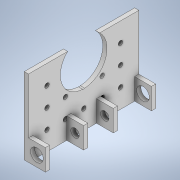
# Autodesk Inventor part: plateForAzimuthKnobs
Saved by Autodesk Inventor 2022.2 (Build 262287010, 287A)
## iProperties
Created: 2022-09-17
Part Number: plateForAzimuthKnobs
Material: Generic
Document SubType Name: Modeling
Designer: robst
Density: 1 g/cm^3
Appearance: Default
Author: robst
Autodesk Inventor part; units mm, degrees
ref_plane "YZ Plane" through (0, 0, 0) normal (1, 0, 0) x (0, 1, 0)
ref_plane "XZ Plane" through (0, 0, 0) normal (0, 1, 0) x (-1, 0, 0)
ref_plane "XY Plane" through (0, 0, 0) normal (0, 0, 1) x (1, 0, 0)
sketch "Sketch1" plane through (0, 0, 0) normal (1, 0, 0) x (0, 1, 0)
  line L0 (-57.2668, 82.55) -> (-57.2668, -82.55)
  line L1 (-57.2668, -82.55) -> (57.2668, -82.55)
  line L2 (57.2668, -82.55) -> (57.2668, 82.55)
  line L3 (57.2668, 82.55) -> (-57.2668, 82.55)
  line L4 (-57.2668, 82.55) -> (57.2668, -82.55) construction
  line L5 (-57.2668, -82.55) -> (57.2668, 82.55) construction
  line L6 (57.2668, 0) -> (-57.2668, 0) construction
  circle A0 centre (31.8668, 0) radius 34.925
  line L7 (-31.8668, 82.55) -> (-31.8668, -82.55) construction
  point P0 (0, 0)
  point P1 (57.2668, -23.9707)
  point P2 (57.2668, 23.9707)
  dimension "d0" = 165.1
  dimension "d1" = 25.4
  dimension "d2" = 69.85
  dimension "d3" = 63.7337
  dimension "d4" = 25.4
  constraints: 16 end point, 4 midpoint, 3 point on line, 2 parallel, 2 perpendicular, 1 centre point, 1 vertical
  measures "d0" distance of L1.end L2.end
  measures "d1" distance from line of A0.centre L2
  measures "d2" diameter of A0
  measures "d3" distance from line of L7 A0.centre
  measures "d4" distance between parallel lines of L7 L0
extrude "Extrusion1" add sketch "Sketch1" against normal blind 6.35 contours L3 L2 A0 L1 L0
sketch "Sketch2" plane through (0, 0, 0) normal (1, 0, 0) x (0, 0, -1)
  line L0 (82.55, -57.2668) -> (-82.55, -57.2668) projected
  line L1 (-82.55, -57.2668) -> (-76.2, -57.2668)
  line L2 (-76.2, -57.2668) -> (-76.2, -25.5168)
  line L3 (-76.2, -25.5168) -> (-82.55, -25.5168)
  line L4 (-82.55, -25.5168) -> (-82.55, -57.2668)
  line L5 (82.55, -57.2668) -> (76.2, -57.2668)
  line L6 (76.2, -57.2668) -> (76.2, -25.5168)
  line L7 (76.2, -25.5168) -> (82.55, -25.5168)
  line L8 (82.55, -25.5168) -> (82.55, -57.2668)
  point P0 (0, 0)
  point P1 (76.2, -57.2668)
  dimension "d7" = 6.35
  dimension "d8" = 6.35
  dimension "d15" = 31.75
  constraints: 16 end point, 4 parallel, 2 horizontal, 2 perpendicular, 1 collinear
  measures "d7" distance between parallel lines of L2 L4
  measures "d8" distance between parallel lines of L6 L8
  measures "d15" distance of L3.end L0.end
extrude "Extrusion2" add sketch "Sketch2" along normal blind 25.2001
sketch "Sketch4" plane through (-6.35, 57.2668, 82.55) normal (0, 0, 1) x (1, 0, 0)
  line L0 (31.5501, -82.7837) -> (31.5501, -114.5337) construction
  line L1 (31.5501, -98.6587) -> (0, -98.6587) construction
  line L2 (0, 0) -> (0, -114.5337) construction
  circle A0 centre (18.8501, -98.6587) radius 9.525
  point P0 (6.35, -57.2668)
  dimension "d11" = 18.8501
  dimension "d12" = 19.05
  constraints: 2 end point, 2 point on line, 1 centre point, 1 horizontal, 1 midpoint
  measures "d11" distance from line of A0.centre L2
  measures "d12" diameter of A0
extrude "Extrusion3" cut sketch "Sketch4" against normal up to surface (6.35 mm away)
sketch "Sketch5" plane through (-6.35, 0, 0) normal (-1, 0, 0) x (0, 0, 1)
  line L0 (-82.55, 57.2668) -> (-82.55, -57.2668) projected
  line L1 (-82.55, -57.2668) -> (82.55, -57.2668) projected
  point P0 (0, 0)
  point P1 (-55.0333, -28.6334)
  dimension "d23" = 27.5167
  dimension "d24" = 28.6334
  measures "d23" distance from line of point (-55.033, -28.633) L0
  measures "d24" distance from line of L1 point (-55.033, -28.633)
hole "Hole1" at (-6.35, -28.6334, -55.0333) direction (1, 0, 0) diameter 6.7564 end through all clearance for "Hex Head Bolt" size "1/4" standard "Ansi Unified Screw Threads"
pattern_linear "Rectangular Pattern1" count 3 spacing 28.6334 along (0, 1, 0) count 5 spacing 27.5167 along (0, 0, 1) of "Hole1"
sketch "Sketch6" plane through (0, 0, 0) normal (1, 0, 0) x (0, 0, -1)
  line L0 (-76.2, -57.2668) -> (76.2, -57.2668) construction
  line L1 (0, -57.2668) -> (0, 0) construction
  line L2 (-82.55, -25.5168) -> (-82.55, -57.2668) construction
  line L3 (82.55, -57.2668) -> (82.55, -25.5168) construction
  line L4 (-82.55, -25.5168) -> (82.55, -25.5168) construction
  line L5 (-19.05, -57.2668) -> (-25.4, -57.2668)
  line L6 (-25.4, -57.2668) -> (-25.4, -25.5168)
  line L7 (-25.4, -25.5168) -> (-19.05, -25.5168)
  line L8 (-19.05, -25.5168) -> (-19.05, -57.2668)
  point P0 (-25.4, -41.3918)
  dimension "d31" = 6.35
  dimension "d32" = 19.05
  constraints: 12 end point, 2 horizontal, 2 midpoint, 2 parallel, 2 point on line, 1 perpendicular, 1 vertical
  measures "d31" distance from line of point (-25.4, -41.392) L8
  measures "d32" distance between parallel lines of L8 L1
extrude "Extrusion4" add sketch "Sketch6" along normal blind 25.2001
sketch "Sketch7" plane through (0, -31.2663, 25.4) normal (0, 0, 1) x (1, 0, 0)
  circle A0 centre (12.5001, -10.1256) radius 6.35
  line L0 (-6.35, 88.5331) -> (-6.35, -26.0006) projected
  point P0 (0, 31.2663)
  dimension "d35" = 12.7
  dimension "d36" = 18.8501
  constraints: 1 centre point
  measures "d35" diameter of A0
  measures "d36" distance from line of A0.centre L0
extrude "Extrusion5" cut sketch "Sketch7" against normal up to surface (6.35 mm away)
mirror "Mirror1" about plane through (0, 0, 0) normal (0, 0, 1) of "Extrusion5", "Extrusion4"
mirror "Mirror2" about plane through (0, 0, 0) normal (0, 0, 1) of "Extrusion3"
equation "\"d0\" = forkWidth"
equation "\"d5\" = wallThickness"
equation "\"d7\" = wallThickness"
equation "\"d8\" = wallThickness"
equation "\"d9\" = centerWormGearAbovePlate + wallThickness"
equation "\"d11\" = centerWormGearAbovePlate"
equation "\"d31\" = wallThickness"
equation "\"d32\" = 0.5 * widthOfWorm"
equation "\"d33\" = centerWormGearAbovePlate + wallThickness"
equation "\"d35\" = holeFor3_8HexShaft"
equation "\"d36\" = centerWormGearAbovePlate"
equation "\"d37\" = centerWormGearAbovePlate + wallThickness"
equation "\"forkWidth\" = 165.1"
equation "\"centerGearToCenterWormGear\" = 73.25868"
equation "\"centerWormGearAbovePlate\" = 18.8501"
equation "\"wallThickness\" = 6.35"
equation "\"widthOfWorm\" = 38.1"
equation "\"holeFor3_8HexShaft\" = 12.7"
body "Solid1"
